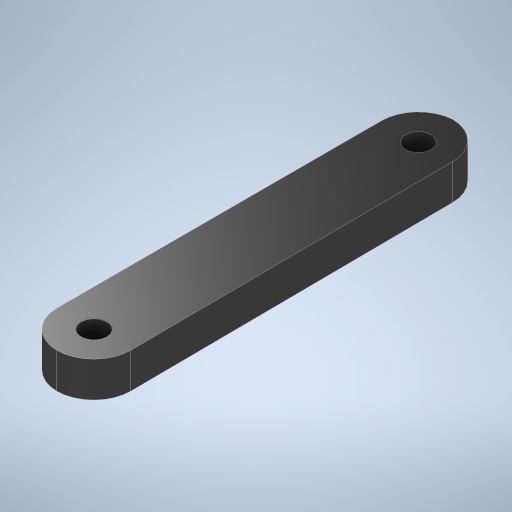
# Autodesk Inventor part: wing bar 2
Saved by Autodesk Inventor 2024.2 (Build 282272000, 272)
## iProperties
Created: 2024-02-08
Part Number: wing bar 2
Material: Generic
Document SubType Name: Modeling
Designer: elite
Density: 1 g/cm^3
Appearance: Glossy - Black
Author: elite
Autodesk Inventor part; units mm, degrees
ref_plane "YZ Plane" through (0, 0, 0) normal (1, 0, 0) x (0, 1, 0)
ref_plane "XZ Plane" through (0, 0, 0) normal (0, 1, 0) x (-1, 0, 0)
ref_plane "XY Plane" through (0, 0, 0) normal (0, 0, 1) x (1, 0, 0)
sketch "Sketch1" plane through (0, 0, 0) normal (0, 1, 0) x (-1, 0, 0)
  line L0 (0, 0) -> (0, -55.88)
  circle A0 centre (0, -55.88) radius 2.2225
  circle A1 centre (0, 0) radius 2.2225
  line L1 (0, 0) -> (0, 6.35)
  line L2 (0, -55.88) -> (0, -62.23)
  line L3 (0, -62.23) -> (6.35, -62.23)
  line L4 (6.35, -62.23) -> (6.35, 6.35)
  line L5 (6.35, 6.35) -> (-6.35, 6.35)
  line L6 (-6.35, 6.35) -> (-5.8392, -62.23)
  line L7 (-5.8392, -62.23) -> (0, -62.23)
  dimension "d0" = 55.88
  dimension "d1" = 4.445
  dimension "d2" = 4.445
  dimension "d3" = 6.35
  dimension "d4" = 6.35
  dimension "d5" = 6.35
  dimension "d6" = 12.7
  dimension "d9" = 6.35
  constraints: 16 end point, 3 horizontal, 3 vertical, 2 centre point, 2 coincident, 1 perpendicular
  measures "d0" distance of L0.start L0.end
  measures "d1" diameter of A0
  measures "d2" diameter of A1
  measures "d3" distance of L1.start L1.end
  measures "d4" distance of L2.start L2.end
  measures "d5" distance of L2.end L3.end
  measures "d6" distance of L4.end L5.end
  measures "d9" distance from line of L0.start L5
extrude "Extrusion1" add sketch "Sketch1" along normal blind 6.096 contours A1 L1 L5 L4 L3 L2 A0 L0 | L0 A0 L2 L7 L6 L5 L1 A1
fillet "Fillet1" radius 6.35 4 edges at (6.35, 3.048, 6.35) (-6.35, 3.048, 6.35) (5.8392, 3.048, -62.23) (-6.35, 3.048, -62.23)
body "Solid1"
